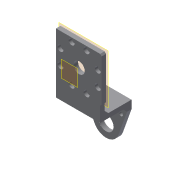
# Autodesk Inventor part: cellSTORM_UC2_Sample_arm_ptycho
Saved by Autodesk Inventor 2019.4 (Build 234330000, 330)
## iProperties
Created: 2020-12-29
Part Number: cellSTORM_UC2_Sample_arm_ptycho
Material: Generic
Document SubType Name: Modeling
Designer: diederichbenedict
Density: 1 g/cm^3
Appearance: Default
Author: diederichbenedict
Autodesk Inventor part; units mm, degrees
ref_plane "YZ Plane" through (0, 0, 0) normal (1, 0, 0) x (0, 1, 0)
ref_plane "XZ Plane" through (0, 0, 0) normal (0, 1, 0) x (-1, 0, 0)
ref_plane "XY Plane" through (0, 0, 0) normal (0, 0, 1) x (1, 0, 0)
ref_plane "Work Plane1" through (0, 0, 0) normal (0, 0, 1) x (1, 0, 0)
sketch "Sketch1" plane through (0, 0, 0) normal (0, 0, 1) x (1, 0, 0)
  circle A0 centre (-10, -25) radius 1.45 projected
  circle A1 centre (-10, 25) radius 1.45 projected
  circle A2 centre (10, 25) radius 1.45 projected
  circle A3 centre (10, -25) radius 1.45 projected
  circle A4 centre (-25, 25) radius 2.325 projected
  circle A5 centre (25, -25) radius 2.325 projected
  circle A6 centre (-25, -25) radius 2.325 projected
  circle A7 centre (25, 25) radius 2.325 projected
  line L0 (28, 30) -> (30, 28) projected
  line L1 (28, 30) -> (-28, 30) projected
  line L2 (-30, 28) -> (-28, 30) projected
  line L3 (-30, 28) -> (-30, -28) projected
  line L4 (-28, -30) -> (-30, -28) projected
  line L5 (-28, -30) -> (28, -30) projected
  line L6 (30, -28) -> (28, -30) projected
  line L7 (30, -28) -> (30, 28) projected
  circle A8 centre (-17.5, -17.5) radius 1.95 projected
  circle A9 centre (17.5, 17.5) radius 1.95 projected
  circle A10 centre (17.5, -17.5) radius 1.95 projected
  circle A11 centre (-17.5, 17.5) radius 1.95 projected
  circle A12 centre (0, 0) radius 7.5 projected
  circle A13 centre (-25.33, -75.26) radius 6.15 projected
  circle A14 centre (25, -10) radius 1.45 projected
  circle A15 centre (-25, -10) radius 1.45 projected
  circle A16 centre (-25, 10) radius 1.45 projected
  circle A17 centre (25, 10) radius 1.45 projected
  line L8 (-28, -30) -> (-31, -30)
  line L9 (-31, -30) -> (-31, 30)
  line L10 (-31, 30) -> (-28, 30)
  line L11 (-28, 30) -> (-28, -30)
  point P0 (0, 0)
  dimension "d0" = 3
  constraints: 8 end point, 2 parallel, 1 horizontal, 1 perpendicular
  measures "d0" distance of L9.end L10.end
extrude "Extrusion1" add sketch "Sketch1" along normal blind 6 contours A4 | A5 | A6 | A7 | L0 L7 L6 L5 L11 L1 | L11 L4 L3 L2 | L2 L3 L4 L8 L9 L10 | A8 | A9 | A10 | A11
ref_plane "Work Plane3" through (0, 0, 19) normal (0, 0, 1) x (1, 0, 0)
sketch "Sketch7" plane through (0, 0, 6) normal (0, 0, 1) x (1, 0, 0)
  circle A0 centre (10, -25) radius 1.45 projected
  circle A1 centre (-10, -25) radius 1.45 projected
  circle A2 centre (-25, -10) radius 1.45 projected
  circle A3 centre (-25, 10) radius 1.45 projected
  circle A4 centre (-10, 25) radius 1.45 projected
  circle A5 centre (10, 25) radius 1.45 projected
  circle A6 centre (25, 10) radius 1.45 projected
  circle A7 centre (25, -10) radius 1.45 projected
  point P0 (0, 0)
hole "Hole1" at (-25, -10, 6) at (-25, 10, 6) at (-10, 25, 6) at (10, 25, 6) at (25, 10, 6) at (25, -10, 6) at (10, -25, 6) at (-10, -25, 6) direction (0, 0, -1) diameter 3.2 end through all counterbore diameter 8 counterbore depth 4
sketch "Sketch10" plane through (-31, -30, 0) normal (-1, 0, 0) x (0, 0, 1)
  line L0 (2, 16) -> (2, 24) projected
  line L1 (0, 0) -> (0, 60) projected
  line L2 (0, 0) -> (6, 0) projected
  line L3 (6, 60) -> (6, 0) projected
  line L4 (0, 60) -> (6, 60) projected
  line L5 (6, 0) -> (6, -20)
  line L6 (6, -20) -> (-30, -20)
  line L7 (-30, -20) -> (-30, -83.2379)
  line L8 (-30, -83.2379) -> (-36, -83.2379)
  line L9 (-36, -83.2379) -> (-36, -14)
  line L10 (-36, -14) -> (0, -14)
  line L11 (0, -14) -> (0, 0)
  line L12 (6, 60) -> (6, 0) projected
  line L13 (0, 0) -> (6, 0)
  point P0 (0, 30)
  dimension "d55" = 20
  dimension "d56" = 90
  dimension "d57" = 6
  dimension "d58" = 90
  dimension "d59" = 90
  dimension "d60" = 90
  dimension "d61" = 30
  dimension "d71" = 6
  constraints: 16 end point, 3 perpendicular, 1 collinear, 1 horizontal, 1 vertical
  measures "d55" distance of L2.end L5.end
  measures "d56" angle of L5 L6
  measures "d57" distance of L7.end L8.end
  measures "d58" angle of L8 L9
  measures "d59" angle of L10 L11
  measures "d60" angle of L9 L10
  measures "d61" distance from line of L1 L6.end
  measures "d71" distance from line of L6 L10.end
extrude "Extrusion9" add sketch "Sketch10" against normal up to surface (59 mm away) contours L2 L5 L6 L7 L8 L9 L10 L11
sketch "Sketch11" plane through (-31, -113.2379, -30) normal (0, 0, 1) x (1, 0, 0)
  line L0 (59, 63.2379) -> (59, 0) projected
  line L1 (0, 63.2379) -> (59, 63.2379) projected
  line L2 (0, 0) -> (0, 63.2379) projected
  line L3 (0, 0) -> (59, 0) projected
  circle A0 centre (31, 31.6189) radius 10
  point P0 (31, 113.2379)
  dimension "d65" = 20
  constraints: 1 centre point
  measures "d65" diameter of A0
extrude "Extrusion10" cut sketch "Sketch11" against normal blind 10 contours A0
chamfer "Chamfer3" distance 5 angle 45 2 edges at (-1.5, -50, -30) (-1.5, -44, 0)
sketch "Sketch12" plane through (-31, -113.2379, -30) normal (0, 0, 1) x (1, 0, 0)
  line L0 (0, 58.2379) -> (59, 58.2379) projected
  line L1 (0, 0) -> (0, 58.2379) projected
  line L2 (0, 0) -> (59, 0) projected
  line L3 (59, 58.2379) -> (59, 0) projected
  circle A0 centre (31, 31.6189) radius 10 projected
  line L4 (51, 51.6189) -> (11, 51.6189)
  line L5 (11, 51.6189) -> (11, 11.6189)
  line L6 (11, 11.6189) -> (51, 11.6189)
  line L7 (51, 11.6189) -> (51, 51.6189)
  line L8 (51, 51.6189) -> (11, 11.6189) construction
  line L9 (11, 51.6189) -> (51, 11.6189) construction
  point P0 (31, 113.2379)
  dimension "d72" = 40
  dimension "d73" = 40
  constraints: 12 end point, 2 midpoint, 2 parallel, 1 horizontal, 1 perpendicular
  measures "d72" distance of L6.end L5.end
  measures "d73" distance of L5.end L4.end
hole "Hole2" at (-20, -101.6189, -30) at (-20, -61.6189, -30) at (20, -61.6189, -30) at (20, -101.6189, -30) direction (0, 0, -1) diameter 4.9 end through all
sketch "Sketch13" plane through (-31, -113.2379, -30) normal (0, 0, 1) x (1, 0, 0)
  circle A0 centre (51, 51.6189) radius 2.45 projected
  circle A1 centre (11, 11.6189) radius 2.45 projected
  circle A2 centre (11, 51.6189) radius 2.45 projected
  circle A3 centre (51, 11.6189) radius 2.45 projected
  line L0 (0, 58.2379) -> (59, 58.2379) projected
  line L1 (0, 0) -> (0, 58.2379) projected
  line L2 (0, 0) -> (59, 0) projected
  line L3 (59, 58.2379) -> (59, 0) projected
  circle A4 centre (31, 31.6189) radius 10 projected
  circle A5 centre (31, 31.6189) radius 17.5
  line L4 (0, 58.2379) -> (15.0116, 24.5041)
  line L5 (0, 58.2379) -> (59, 58.2379) projected
  line L6 (59, 58.2379) -> (47.4948, 25.7733)
  point P0 (31, 113.2379)
  dimension "d81" = 35
  constraints: 4 end point, 2 point on circle, 2 tangent, 1 centre point, 1 coincident
  measures "d81" diameter of A5
extrude "Extrusion11" cut sketch "Sketch13" against normal through all contours L4 A5 L6 L3 L2 L1
equation "\"d57\" = d1"
equation "\"d71\" = d1"
equation "\"d1\" = 6"
body "Solid1"
